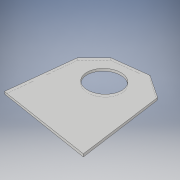
# Autodesk Inventor part: Crossbeam Bearing Mount
Saved by Autodesk Inventor 2019 (Build 230136000, 136)
## iProperties
Created: 2018-09-28
Part Number: Crossbeam Bearing Mount
Material: Generic
Document SubType Name: Modeling
Designer: Adhik
Density: 1 g/cm^3
Appearance: Default
Mass: 3.73695 g
Surface Area: 51.3793 cm^2
Volume: 3.73695 cm^3
Author: Adhik
Autodesk Inventor part; units mm, degrees
ref_plane "YZ Plane" through (0, 0, 0) normal (1, 0, 0) x (0, 1, 0)
ref_plane "XZ Plane" through (0, 0, 0) normal (0, 1, 0) x (-1, 0, 0)
ref_plane "XY Plane" through (0, 0, 0) normal (0, 0, 1) x (1, 0, 0)
sketch "Sketch1" plane through (0, 0, 0) normal (0, 1, 0) x (-1, 0, 0)
  line L0 (0, -40.005) -> (0, 40.005) construction
  line L1 (35.56, 0) -> (-35.56, 0) construction
  line L2 (25.4, -28.575) -> (-25.4, -28.575)
  line L3 (-25.4, -28.575) -> (-25.4, 28.575)
  line L4 (-25.4, 28.575) -> (25.4, 28.575)
  line L5 (25.4, 28.575) -> (25.4, -28.575)
  circle A0 centre (0, -9.525) radius 11.1125
  line L6 (25.4, 3.175) -> (-25.4, 3.175) construction
  circle A1 centre (0, -9.525) radius 12.7 construction
  point P0 (0, 0)
  point P1 (0, 28.575)
  point P2 (25.4, 0)
  dimension "d0" = 25.4
  dimension "d1" = 22.225
  dimension "d2" = 25.4
  dimension "d3" = 57.15
  dimension "d4" = 50.8
  constraints: 10 end point, 5 point on line, 2 centre point, 2 midpoint, 2 parallel, 2 perpendicular, 1 coincident, 1 horizontal, 1 tangent
  measures "d0" distance between parallel lines of L4 L6
  measures "d1" diameter of A0
  measures "d2" diameter of A1
  measures "d3" distance of L2.end L3.end
  measures "d4" distance of L3.end L4.end
extrude "Extrusion1" add sketch "Sketch1" along normal blind 1.5875
chamfer "Chamfer1" distance 12.7 angle 45 2 edges at (-25.4, 0.7937, -28.575) (25.4, 0.7937, -28.575)
body "Solid1"
